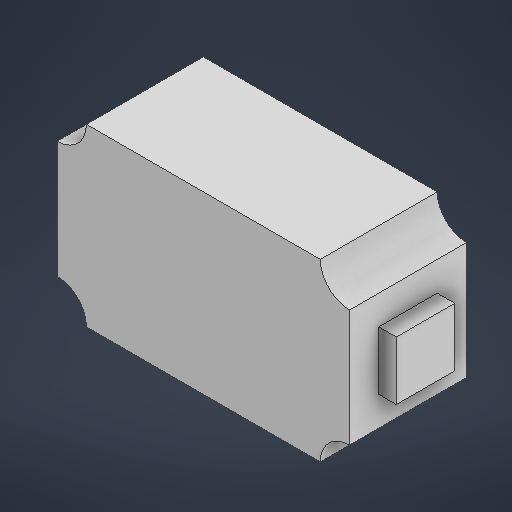
# Autodesk Inventor part: receptor ftth fibra
Saved by Autodesk Inventor 2026.2 (Build 302298010, 298A)
## iProperties
Created: 2026-04-26
Part Number: receptor ftth fibra
Material: Genérico
Document SubType Name: Modeling
Designer: Lucas David
Density: 1 g/cm^3
Appearance: Padrão
Author: Lucas David
Autodesk Inventor part; units mm, degrees
ref_plane "YZ Plane" through (0, 0, 0) normal (1, 0, 0) x (0, 1, 0)
ref_plane "XZ Plane" through (0, 0, 0) normal (0, 1, 0) x (-1, 0, 0)
ref_plane "XY Plane" through (0, 0, 0) normal (0, 0, 1) x (1, 0, 0)
sketch "Esboço1" plane through (0, 0, 0) normal (0, 0, 1) x (1, 0, 0)
  line L0 (-20, -15) -> (20, -15)
  line L1 (25, -10) -> (25, 10)
  line L2 (20, 15) -> (-20, 15)
  line L3 (-25, 10) -> (-25, -10)
  line L4 (-25, -15) -> (25, 15) construction
  line L5 (10.842, 0) -> (-10.842, 0) construction
  line L6 (0, 2.6199) -> (0, -2.6199) construction
  line L7 (1.3987, 0) -> (-1.3987, 0) construction
  arc A0 (20, 15) -> (25, 10) centre (25, 15) ccw
  arc A1 (25, -10) -> (20, -15) centre (25, -15) ccw
  arc A2 (-25, 10) -> (-20, 15) centre (-25, 15) ccw
  arc A3 (-20, -15) -> (-25, -10) centre (-25, -15) ccw
  point P0 (0, 0)
  dimension "d0" = 30
  dimension "d1" = 50
  dimension "d22" = 10
  dimension "d23" = 5
  dimension "d24" = 5
  constraints: 16 end point, 8 point on circle, 8 symmetric about line, 4 centre point, 4 midpoint, 3 horizontal, 2 parallel, 1 coincident, 1 perpendicular, 1 vertical, 3 other
  measures "d0" distance between parallel lines of L0 L2
  measures "d1" distance between parallel lines of L1 L3
  measures "d22" diameter of A0
  measures "d23" distance from line of L1 L2.start
  measures "d24" distance from line of L2 L1.end
extrude "Extrusão1" add sketch "Esboço1" along normal blind 20
sketch "Esboço2" plane through (-25, -10, 0) normal (-1, 0, 0) x (0, 0, 1)
  circle A0 centre (10, 8) radius 2.5
  line L0 (20, 20) -> (20, 0) projected
  line L1 (0, 0) -> (20, 0) projected
  circle A1 centre (10, 8) radius 3.5
  line L2 (10, 0) -> (10, 11.9886) construction
  line L3 (0, -5) -> (20, -5) projected
  point P0 (0, 10)
  dimension "d10" = 1
  dimension "d25" = 5
  dimension "d27" = 8
  constraints: 2 centre point, 2 end point, 1 midpoint, 1 point on line, 1 vertical
  measures "d10" radial gap between concentric circles of A0 A1
  measures "d25" diameter of A0
  measures "d27" distance from line of L1 A0.centre
extrude "Extrusão2" add sketch "Esboço2" along normal blind 2
extrude "Extrusão3" add sketch "Esboço2" along normal blind 5 contours A0
fillet "Arredondamento1" radius 1 1 edges at (-27, -2, 6.5)
thread "Rosca1" size "M2x0.4" class "6g" standard "ANSI Metric M Profile" full length
sketch "Esboço5" plane through (25, -10, 0) normal (1, 0, 0) x (0, 0, -1)
  line L0 (-20, 20) -> (0, 20) projected
  line L1 (0, 20) -> (0, 0) projected
  line L2 (0, 0) -> (-20, 0) projected
  line L3 (-20, 0) -> (-20, 20) projected
  line L4 (-15, 15) -> (-5, 15)
  line L5 (-5, 15) -> (-5, 5)
  line L6 (-5, 5) -> (-15, 5)
  line L7 (-15, 5) -> (-15, 15)
  point P0 (0, 10)
  dimension "d28" = 5
  constraints: 8 end point, 3 other
  measures "d28" distance between parallel lines of L0 L4
extrude "Extrusão4" add sketch "Esboço5" along normal blind 3 contours L4 L5 L6 L7
